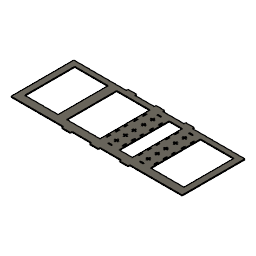
Plaat (Autodesk Fusion 360 design; units mm, degrees)
part number: 2026-03-19-08-41-09-141
Autodesk Fusion 360 part; units mm, degrees
sketch "Sketch1" plane through (0, 0, 0) normal (0, 0, 1) x (1, 0, 0)
  line L0 (-877.2181, -324.1666) -> (-877.2181, 35.8334)
  line L1 (-301.7378, 5.8334) -> (-226.7378, 5.8334)
  line L2 (-226.7378, 5.8334) -> (-226.7378, -279.1666)
  line L3 (-226.7378, -279.1666) -> (-301.7378, -279.1666)
  line L4 (-301.7378, -279.1666) -> (-301.7378, 5.8334)
  line L5 (-122.2181, 5.8334) -> (-122.2181, -279.1666)
  line L6 (67.7819, 5.8334) -> (-122.2181, 5.8334)
  line L7 (-652.2181, -279.1666) -> (-652.2181, 5.8334)
  line L8 (-842.2181, -279.1666) -> (-652.2181, -279.1666)
  line L9 (-652.2181, 5.8334) -> (-842.2181, 5.8334)
  line L10 (-842.2181, 5.8334) -> (-842.2181, -279.1666)
  line L11 (-412.2181, -279.1666) -> (-412.2181, 5.8334)
  line L12 (-602.2181, 5.8334) -> (-602.2181, -279.1666)
  line L13 (102.7819, 35.8334) -> (102.7819, -324.1666)
  line L14 (-358.9778, -149.6866) -> (-354.9778, -149.6866)
  line L15 (-354.9778, -129.6866) -> (-358.9778, -129.6866)
  line L16 (-366.9778, -137.6866) -> (-366.9778, -141.6866)
  line L17 (-358.9778, -137.6866) -> (-366.9778, -137.6866)
  line L18 (-346.9778, -137.6866) -> (-354.9778, -137.6866)
  line L19 (-358.9778, -141.6866) -> (-358.9778, -149.6866)
  line L20 (-354.9778, -149.6866) -> (-354.9778, -141.6866)
  line L21 (-366.9778, -141.6866) -> (-358.9778, -141.6866)
  line L22 (-346.9778, -141.6866) -> (-346.9778, -137.6866)
  line L23 (-358.9778, -129.6866) -> (-358.9778, -137.6866)
  line L24 (-354.9778, -137.6866) -> (-354.9778, -129.6866)
  line L25 (-354.9778, -141.6866) -> (-346.9778, -141.6866)
  line L26 (-354.9778, -31.3266) -> (-354.9778, -23.3266)
  line L27 (-346.9778, -35.3266) -> (-346.9778, -31.3266)
  line L28 (-354.9778, -43.3266) -> (-354.9778, -35.3266)
  line L29 (-358.9778, -31.3266) -> (-366.9778, -31.3266)
  line L30 (-358.9778, -23.3266) -> (-358.9778, -31.3266)
  line L31 (-358.9778, -35.3266) -> (-358.9778, -43.3266)
  line L32 (-358.9778, -43.3266) -> (-354.9778, -43.3266)
  line L33 (-346.9778, -31.3266) -> (-354.9778, -31.3266)
  line L34 (-354.9778, -23.3266) -> (-358.9778, -23.3266)
  line L35 (-366.9778, -35.3266) -> (-358.9778, -35.3266)
  line L36 (-354.9778, -35.3266) -> (-346.9778, -35.3266)
  line L37 (-366.9778, -31.3266) -> (-366.9778, -35.3266)
  line L38 (-358.9778, -94.4866) -> (-354.9778, -94.4866)
  line L39 (-354.9778, -82.4866) -> (-354.9778, -74.4866)
  line L40 (-354.9778, -74.4866) -> (-358.9778, -74.4866)
  line L41 (-354.9778, -86.4866) -> (-346.9778, -86.4866)
  line L42 (-346.9778, -86.4866) -> (-346.9778, -82.4866)
  line L43 (-358.9778, -86.4866) -> (-358.9778, -94.4866)
  line L44 (-366.9778, -86.4866) -> (-358.9778, -86.4866)
  line L45 (-366.9778, -82.4866) -> (-366.9778, -86.4866)
  line L46 (-354.9778, -94.4866) -> (-354.9778, -86.4866)
  line L47 (-346.9778, -82.4866) -> (-354.9778, -82.4866)
  line L48 (-358.9778, -82.4866) -> (-366.9778, -82.4866)
  line L49 (-358.9778, -74.4866) -> (-358.9778, -82.4866)
  line L50 (-358.9778, -238.0066) -> (-366.9778, -238.0066)
  line L51 (-354.9778, -238.0066) -> (-354.9778, -230.0066)
  line L52 (-366.9778, -238.0066) -> (-366.9778, -242.0066)
  line L53 (-354.9778, -242.0066) -> (-346.9778, -242.0066)
  line L54 (-358.9778, -230.0066) -> (-358.9778, -238.0066)
  line L55 (-358.9778, -242.0066) -> (-358.9778, -250.0066)
  line L56 (-358.9778, -250.0066) -> (-354.9778, -250.0066)
  line L57 (-346.9778, -242.0066) -> (-346.9778, -238.0066)
  line L58 (-346.9778, -238.0066) -> (-354.9778, -238.0066)
  line L59 (-366.9778, -242.0066) -> (-358.9778, -242.0066)
  line L60 (-354.9778, -250.0066) -> (-354.9778, -242.0066)
  line L61 (-354.9778, -230.0066) -> (-358.9778, -230.0066)
  line L62 (-354.9778, -190.8466) -> (-346.9778, -190.8466)
  line L63 (-366.9778, -186.8466) -> (-366.9778, -190.8466)
  line L64 (-358.9778, -190.8466) -> (-358.9778, -198.8466)
  line L65 (-358.9778, -198.8466) -> (-354.9778, -198.8466)
  line L66 (-354.9778, -186.8466) -> (-354.9778, -178.8466)
  line L67 (-346.9778, -186.8466) -> (-354.9778, -186.8466)
  line L68 (-358.9778, -186.8466) -> (-366.9778, -186.8466)
  line L69 (-366.9778, -190.8466) -> (-358.9778, -190.8466)
  line L70 (-354.9778, -178.8466) -> (-358.9778, -178.8466)
  line L71 (-346.9778, -190.8466) -> (-346.9778, -186.8466)
  line L72 (-354.9778, -198.8466) -> (-354.9778, -190.8466)
  line L73 (-358.9778, -178.8466) -> (-358.9778, -186.8466)
  line L74 (-356.9778, -139.6866) -> (-357.8185, -139.6866) construction
  line L75 (-357.8185, -139.6866) -> (-358.9778, -139.6866) construction
  line L76 (-602.2181, -279.1666) -> (-580.1685, -279.1666)
  line L77 (-580.1685, -279.1666) -> (-412.2181, -279.1666)
  line L78 (-602.2181, 5.8334) -> (-412.2181, 5.8334)
  line L79 (-122.2181, -279.1666) -> (67.7819, -279.1666)
  line L80 (67.7819, -279.1666) -> (67.7819, 5.8334)
  line L81 (-527.2181, 35.8334) -> (-527.2181, 45.8334)
  line L82 (-527.2181, 45.8334) -> (-577.2181, 45.8334)
  line L83 (-577.2181, 45.8334) -> (-577.2181, 35.8334)
  line L84 (-400.2181, -23.3266) -> (-404.2181, -23.3266)
  line L85 (-404.2181, -23.3266) -> (-404.2181, -43.3266)
  line L86 (-404.2181, -43.3266) -> (-400.2181, -43.3266)
  line L87 (-400.2181, -43.3266) -> (-400.2181, -23.3266)
  line L88 (-400.2181, -74.4866) -> (-404.2181, -74.4866)
  line L89 (-404.2181, -74.4866) -> (-404.2181, -94.4866)
  line L90 (-404.2181, -94.4866) -> (-400.2181, -94.4866)
  line L91 (-400.2181, -94.4866) -> (-400.2181, -74.4866)
  line L92 (-400.2181, -132.7485) -> (-404.2181, -132.7485)
  line L93 (-404.2181, -132.7485) -> (-404.2181, -149.6866)
  line L94 (-404.2181, -149.6866) -> (-400.2181, -149.6866)
  line L95 (-400.2181, -149.6866) -> (-400.2181, -132.7485)
  line L96 (-400.2181, -178.8466) -> (-404.2181, -178.8466)
  line L97 (-404.2181, -178.8466) -> (-404.2181, -198.8466)
  line L98 (-404.2181, -198.8466) -> (-400.2181, -198.8466)
  line L99 (-400.2181, -198.8466) -> (-400.2181, -178.8466)
  line L100 (-400.2181, -230.0066) -> (-404.2181, -230.0066)
  line L101 (-404.2181, -230.0066) -> (-404.2181, -250.0066)
  line L102 (-404.2181, -250.0066) -> (-400.2181, -250.0066)
  line L103 (-400.2181, -250.0066) -> (-400.2181, -230.0066)
  line L104 (-309.7378, -230.0066) -> (-313.7378, -230.0066)
  line L105 (-313.7378, -230.0066) -> (-313.7378, -250.0066)
  line L106 (-313.7378, -250.0066) -> (-309.7378, -250.0066)
  line L107 (-309.7378, -250.0066) -> (-309.7378, -230.0066)
  line L108 (-309.7378, -178.8466) -> (-313.7378, -178.8466)
  line L109 (-313.7378, -178.8466) -> (-313.7378, -198.8466)
  line L110 (-313.7378, -198.8466) -> (-309.7378, -198.8466)
  line L111 (-309.7378, -198.8466) -> (-309.7378, -178.8466)
  line L112 (-309.7378, -132.7485) -> (-313.7378, -132.7485)
  line L113 (-313.7378, -132.7485) -> (-313.7378, -149.6866)
  line L114 (-313.7378, -149.6866) -> (-309.7378, -149.6866)
  line L115 (-309.7378, -149.6866) -> (-309.7378, -132.7485)
  line L116 (-309.7378, -74.4866) -> (-313.7378, -74.4866)
  line L117 (-313.7378, -74.4866) -> (-313.7378, -94.4866)
  line L118 (-313.7378, -94.4866) -> (-309.7378, -94.4866)
  line L119 (-309.7378, -94.4866) -> (-309.7378, -74.4866)
  line L120 (-309.7378, -23.3266) -> (-313.7378, -23.3266)
  line L121 (-313.7378, -23.3266) -> (-313.7378, -43.3266)
  line L122 (-313.7378, -43.3266) -> (-309.7378, -43.3266)
  line L123 (-309.7378, -43.3266) -> (-309.7378, -23.3266)
  line L124 (-197.2181, 35.8334) -> (-197.2181, 45.8334)
  line L125 (-197.2181, 45.8334) -> (-247.2181, 45.8334)
  line L126 (-247.2181, 45.8334) -> (-247.2181, 35.8334)
  line L127 (-367.2181, 35.8334) -> (-367.2181, 45.8334)
  line L128 (-367.2181, 45.8334) -> (-417.2181, 45.8334)
  line L129 (-417.2181, 45.8334) -> (-417.2181, 35.8334)
  line L130 (-877.2181, 35.8334) -> (-577.2181, 35.8334)
  line L131 (-527.2181, 35.8334) -> (-417.2181, 35.8334)
  line L132 (-367.2181, 35.8334) -> (-247.2181, 35.8334)
  line L133 (-197.2181, 35.8334) -> (102.7819, 35.8334)
  line L134 (-366.9778, -279.1666) -> (-346.9778, -279.1666)
  line L135 (-346.9778, -279.1666) -> (-346.9778, -275.1666)
  line L136 (-346.9778, -275.1666) -> (-366.9778, -275.1666)
  line L137 (-366.9778, -275.1666) -> (-366.9778, -279.1666)
  line L138 (-366.9778, 5.8334) -> (-346.9778, 5.8334)
  line L139 (-346.9778, 5.8334) -> (-346.9778, 1.8334)
  line L140 (-346.9778, 1.8334) -> (-366.9778, 1.8334)
  line L141 (-366.9778, 1.8334) -> (-366.9778, 5.8334)
  line L142 (-527.2181, -324.1666) -> (-527.2181, -334.1666)
  line L143 (-527.2181, -334.1666) -> (-577.2181, -334.1666)
  line L144 (-577.2181, -334.1666) -> (-577.2181, -324.1666)
  line L145 (-367.2181, -324.1666) -> (-367.2181, -334.1666)
  line L146 (-367.2181, -334.1666) -> (-417.2181, -334.1666)
  line L147 (-417.2181, -334.1666) -> (-417.2181, -324.1666)
  line L148 (-197.2181, -324.1666) -> (-197.2181, -334.1666)
  line L149 (-197.2181, -334.1666) -> (-247.2181, -334.1666)
  line L150 (-247.2181, -334.1666) -> (-247.2181, -324.1666)
  line L151 (-877.2181, -324.1666) -> (-577.2181, -324.1666)
  line L152 (-527.2181, -324.1666) -> (-417.2181, -324.1666)
  line L153 (-367.2181, -324.1666) -> (-247.2181, -324.1666)
  line L154 (-197.2181, -324.1666) -> (102.7819, -324.1666)
  line L155 (-127.7378, -178.8466) -> (-131.7378, -178.8466)
  line L156 (-127.7378, -250.0066) -> (-127.7378, -230.0066)
  line L157 (-127.7378, -198.8466) -> (-127.7378, -178.8466)
  line L158 (-131.7378, -198.8466) -> (-127.7378, -198.8466)
  line L159 (-131.7378, -230.0066) -> (-131.7378, -250.0066)
  line L160 (-131.7378, -178.8466) -> (-131.7378, -198.8466)
  line L161 (-127.7378, -230.0066) -> (-131.7378, -230.0066)
  line L162 (-131.7378, -250.0066) -> (-127.7378, -250.0066)
  line L163 (-127.7378, -149.6866) -> (-127.7378, -132.7485)
  line L164 (-127.7378, -94.4866) -> (-127.7378, -74.4866)
  line L165 (-131.7378, -132.7485) -> (-131.7378, -149.6866)
  line L166 (-131.7378, -74.4866) -> (-131.7378, -94.4866)
  line L167 (-127.7378, -74.4866) -> (-131.7378, -74.4866)
  line L168 (-127.7378, -132.7485) -> (-131.7378, -132.7485)
  line L169 (-131.7378, -149.6866) -> (-127.7378, -149.6866)
  line L170 (-131.7378, -94.4866) -> (-127.7378, -94.4866)
  line L171 (-127.7378, -43.3266) -> (-127.7378, -23.3266)
  line L172 (-131.7378, -23.3266) -> (-131.7378, -43.3266)
  line L173 (-131.7378, -43.3266) -> (-127.7378, -43.3266)
  line L174 (-127.7378, -23.3266) -> (-131.7378, -23.3266)
  line L175 (-184.9778, -279.1666) -> (-164.9778, -279.1666)
  line L176 (-172.9778, -198.8466) -> (-172.9778, -190.8466)
  line L177 (-218.2181, -132.7485) -> (-222.2181, -132.7485)
  line L178 (-184.9778, -190.8466) -> (-176.9778, -190.8466)
  line L179 (-184.9778, -186.8466) -> (-184.9778, -190.8466)
  line L180 (-175.8185, -139.6866) -> (-176.9778, -139.6866) construction
  line L181 (-164.9778, -279.1666) -> (-164.9778, -275.1666)
  line L182 (-172.9778, -149.6866) -> (-172.9778, -141.6866)
  line L183 (-176.9778, -242.0066) -> (-176.9778, -250.0066)
  line L184 (-172.9778, -230.0066) -> (-176.9778, -230.0066)
  line L185 (-218.2181, -178.8466) -> (-222.2181, -178.8466)
  line L186 (-184.9778, -275.1666) -> (-184.9778, -279.1666)
  line L187 (-176.9778, -82.4866) -> (-184.9778, -82.4866)
  line L188 (-176.9778, -137.6866) -> (-184.9778, -137.6866)
  line L189 (-172.9778, -250.0066) -> (-172.9778, -242.0066)
  line L190 (-172.9778, -190.8466) -> (-164.9778, -190.8466)
  line L191 (-218.2181, -230.0066) -> (-222.2181, -230.0066)
  line L192 (-164.9778, -141.6866) -> (-164.9778, -137.6866)
  line L193 (-172.9778, -178.8466) -> (-176.9778, -178.8466)
  line L194 (-164.9778, -86.4866) -> (-164.9778, -82.4866)
  line L195 (-222.2181, -178.8466) -> (-222.2181, -198.8466)
  line L196 (-164.9778, -275.1666) -> (-184.9778, -275.1666)
  line L197 (-164.9778, -242.0066) -> (-164.9778, -238.0066)
  line L198 (-218.2181, -149.6866) -> (-218.2181, -132.7485)
  line L199 (-164.9778, 1.8334) -> (-184.9778, 1.8334)
  line L200 (-164.9778, -31.3266) -> (-172.9778, -31.3266)
  line L201 (-184.9778, -35.3266) -> (-176.9778, -35.3266)
  line L202 (-172.9778, -137.6866) -> (-172.9778, -129.6866)
  line L203 (-184.9778, -82.4866) -> (-184.9778, -86.4866)
  line L204 (-164.9778, -82.4866) -> (-172.9778, -82.4866)
  line L205 (-222.2181, -94.4866) -> (-218.2181, -94.4866)
  line L206 (-172.9778, -74.4866) -> (-176.9778, -74.4866)
  line L207 (-222.2181, -74.4866) -> (-222.2181, -94.4866)
  line L208 (-172.9778, -94.4866) -> (-172.9778, -86.4866)
  line L209 (-164.9778, -137.6866) -> (-172.9778, -137.6866)
  line L210 (-164.9778, -35.3266) -> (-164.9778, -31.3266)
  line L211 (-176.9778, -35.3266) -> (-176.9778, -43.3266)
  line L212 (-172.9778, -82.4866) -> (-172.9778, -74.4866)
  line L213 (-172.9778, -86.4866) -> (-164.9778, -86.4866)
  line L214 (-184.9778, 5.8334) -> (-164.9778, 5.8334)
  line L215 (-218.2181, -43.3266) -> (-218.2181, -23.3266)
  line L216 (-164.9778, 5.8334) -> (-164.9778, 1.8334)
  line L217 (-176.9778, -129.6866) -> (-176.9778, -137.6866)
  line L218 (-176.9778, -31.3266) -> (-184.9778, -31.3266)
  line L219 (-184.9778, -141.6866) -> (-176.9778, -141.6866)
  line L220 (-184.9778, -31.3266) -> (-184.9778, -35.3266)
  line L221 (-176.9778, -23.3266) -> (-176.9778, -31.3266)
  line L222 (-172.9778, -129.6866) -> (-176.9778, -129.6866)
  line L223 (-176.9778, -94.4866) -> (-172.9778, -94.4866)
  line L224 (-164.9778, -190.8466) -> (-164.9778, -186.8466)
  line L225 (-164.9778, -238.0066) -> (-172.9778, -238.0066)
  line L226 (-172.9778, -35.3266) -> (-164.9778, -35.3266)
  line L227 (-222.2181, -132.7485) -> (-222.2181, -149.6866)
  line L228 (-172.9778, -186.8466) -> (-172.9778, -178.8466)
  line L229 (-222.2181, -198.8466) -> (-218.2181, -198.8466)
  line L230 (-184.9778, -86.4866) -> (-176.9778, -86.4866)
  line L231 (-184.9778, -137.6866) -> (-184.9778, -141.6866)
  line L232 (-172.9778, -141.6866) -> (-164.9778, -141.6866)
  line L233 (-218.2181, -23.3266) -> (-222.2181, -23.3266)
  line L234 (-184.9778, 1.8334) -> (-184.9778, 5.8334)
  line L235 (-172.9778, -242.0066) -> (-164.9778, -242.0066)
  line L236 (-176.9778, -149.6866) -> (-172.9778, -149.6866)
  line L237 (-184.9778, -238.0066) -> (-184.9778, -242.0066)
  line L238 (-222.2181, -250.0066) -> (-218.2181, -250.0066)
  line L239 (-176.9778, -178.8466) -> (-176.9778, -186.8466)
  line L240 (-222.2181, -230.0066) -> (-222.2181, -250.0066)
  line L241 (-172.9778, -31.3266) -> (-172.9778, -23.3266)
  line L242 (-176.9778, -190.8466) -> (-176.9778, -198.8466)
  line L243 (-176.9778, -141.6866) -> (-176.9778, -149.6866)
  line L244 (-172.9778, -238.0066) -> (-172.9778, -230.0066)
  line L245 (-176.9778, -250.0066) -> (-172.9778, -250.0066)
  line L246 (-176.9778, -186.8466) -> (-184.9778, -186.8466)
  line L247 (-174.9778, -139.6866) -> (-175.8185, -139.6866) construction
  line L248 (-164.9778, -186.8466) -> (-172.9778, -186.8466)
  line L249 (-172.9778, -43.3266) -> (-172.9778, -35.3266)
  line L250 (-172.9778, -23.3266) -> (-176.9778, -23.3266)
  line L251 (-176.9778, -86.4866) -> (-176.9778, -94.4866)
  line L252 (-184.9778, -242.0066) -> (-176.9778, -242.0066)
  line L253 (-218.2181, -198.8466) -> (-218.2181, -178.8466)
  line L254 (-176.9778, -238.0066) -> (-184.9778, -238.0066)
  line L255 (-218.2181, -250.0066) -> (-218.2181, -230.0066)
  line L256 (-176.9778, -43.3266) -> (-172.9778, -43.3266)
  line L257 (-176.9778, -198.8466) -> (-172.9778, -198.8466)
  line L258 (-218.2181, -94.4866) -> (-218.2181, -74.4866)
  line L259 (-222.2181, -149.6866) -> (-218.2181, -149.6866)
  line L260 (-176.9778, -230.0066) -> (-176.9778, -238.0066)
  line L261 (-176.9778, -74.4866) -> (-176.9778, -82.4866)
  line L262 (-218.2181, -74.4866) -> (-222.2181, -74.4866)
  line L263 (-222.2181, -43.3266) -> (-218.2181, -43.3266)
  line L264 (-222.2181, -23.3266) -> (-222.2181, -43.3266)
  point P0 (-356.9778, -139.6866)
  point P1 (-358.9778, -139.6866)
  point P2 (-174.9778, -139.6866)
  point P3 (-176.9778, -139.6866)
  constraint vertical L11
  constraint horizontal L14
  constraint perpendicular L14 L20
  constraint perpendicular L20 L25
  constraint perpendicular L22 L25
  constraint perpendicular L18 L22
  constraint perpendicular L18 L24
  constraint perpendicular L15 L24
  constraint perpendicular L18 L23
  constraint perpendicular L17 L23
  constraint perpendicular L16 L17
  constraint perpendicular L16 L21
  constraint perpendicular L19 L21
  constraint horizontal L32
  constraint perpendicular L28 L32
  constraint perpendicular L28 L36
  constraint perpendicular L27 L36
  constraint perpendicular L27 L33
  constraint perpendicular L26 L33
  constraint perpendicular L26 L34
  constraint perpendicular L30 L33
  constraint perpendicular L29 L30
  constraint perpendicular L29 L37
  constraint perpendicular L35 L37
  constraint perpendicular L31 L35
  constraint horizontal L38
  constraint perpendicular L38 L46
  constraint perpendicular L41 L46
  constraint perpendicular L41 L42
  constraint perpendicular L42 L47
  constraint perpendicular L39 L47
  constraint perpendicular L39 L40
  constraint perpendicular L47 L49
  constraint perpendicular L48 L49
  constraint perpendicular L45 L48
  constraint perpendicular L44 L45
  constraint perpendicular L43 L44
  constraint horizontal L56
  constraint perpendicular L56 L60
  constraint perpendicular L53 L60
  constraint perpendicular L53 L57
  constraint perpendicular L57 L58
  constraint perpendicular L51 L58
  constraint perpendicular L51 L61
  constraint perpendicular L54 L58
  constraint perpendicular L50 L54
  constraint perpendicular L50 L52
  constraint perpendicular L52 L59
  constraint perpendicular L55 L59
  constraint horizontal L65
  constraint perpendicular L65 L72
  constraint perpendicular L62 L72
  constraint perpendicular L62 L71
  constraint perpendicular L67 L71
  constraint perpendicular L66 L67
  constraint perpendicular L66 L70
  constraint perpendicular L67 L73
  constraint perpendicular L68 L73
  constraint perpendicular L63 L68
  constraint perpendicular L63 L69
  constraint perpendicular L64 L69
  constraint coincident P0 L74.start
  constraint coincident P1 L75.end
  constraint perpendicular L12 L76
  constraint perpendicular L11 L77
  constraint perpendicular L11 L78
  constraint perpendicular L5 L79
  constraint perpendicular L6 L80
  constraint vertical L81
  constraint horizontal L82
  constraint vertical L83
  constraint horizontal L84
  constraint vertical L85
  constraint horizontal L86
  constraint vertical L87
  constraint horizontal L88
  constraint vertical L89
  constraint horizontal L90
  constraint vertical L91
  constraint horizontal L92
  constraint vertical L93
  constraint horizontal L94
  constraint vertical L95
  constraint horizontal L96
  constraint vertical L97
  constraint horizontal L98
  constraint vertical L99
  constraint horizontal L100
  constraint vertical L101
  constraint horizontal L102
  constraint vertical L103
  constraint horizontal L104
  constraint vertical L105
  constraint horizontal L106
  constraint vertical L107
  constraint horizontal L108
  constraint vertical L109
  constraint horizontal L110
  constraint vertical L111
  constraint horizontal L112
  constraint vertical L113
  constraint horizontal L114
  constraint vertical L115
  constraint horizontal L116
  constraint vertical L117
  constraint horizontal L118
  constraint vertical L119
  constraint horizontal L120
  constraint vertical L121
  constraint horizontal L122
  constraint vertical L123
  constraint vertical L124
  constraint horizontal L125
  constraint vertical L126
  constraint vertical L127
  constraint horizontal L128
  constraint vertical L129
  constraint perpendicular L83 L130
  constraint perpendicular L129 L131
  constraint perpendicular L126 L132
  constraint perpendicular L13 L133
  constraint horizontal L134
  constraint vertical L135
  constraint horizontal L136
  constraint vertical L137
  constraint horizontal L138
  constraint vertical L139
  constraint horizontal L140
  constraint vertical L141
  constraint vertical L142
  constraint horizontal L143
  constraint vertical L144
  constraint vertical L145
  constraint horizontal L146
  constraint vertical L147
  constraint vertical L148
  constraint horizontal L149
  constraint vertical L150
  constraint perpendicular L150 L153
  constraint perpendicular L13 L154
  constraint horizontal L236
  constraint perpendicular L182 L236
  constraint perpendicular L182 L232
  constraint perpendicular L192 L232
  constraint perpendicular L192 L209
  constraint perpendicular L202 L209
  constraint perpendicular L202 L222
  constraint perpendicular L209 L217
  constraint perpendicular L188 L217
  constraint perpendicular L188 L231
  constraint perpendicular L219 L231
  constraint perpendicular L219 L243
  constraint horizontal L256
  constraint perpendicular L249 L256
  constraint perpendicular L226 L249
  constraint perpendicular L210 L226
  constraint perpendicular L200 L210
  constraint perpendicular L200 L241
  constraint perpendicular L241 L250
  constraint perpendicular L200 L221
  constraint perpendicular L218 L221
  constraint perpendicular L218 L220
  constraint perpendicular L201 L220
  constraint perpendicular L201 L211
  constraint horizontal L223
  constraint perpendicular L208 L223
  constraint perpendicular L208 L213
  constraint perpendicular L194 L213
  constraint perpendicular L194 L204
  constraint perpendicular L204 L212
  constraint perpendicular L206 L212
  constraint perpendicular L204 L261
  constraint perpendicular L187 L261
  constraint perpendicular L187 L203
  constraint perpendicular L203 L230
  constraint perpendicular L230 L251
  constraint horizontal L245
  constraint perpendicular L189 L245
  constraint perpendicular L189 L235
  constraint perpendicular L197 L235
  constraint perpendicular L197 L225
  constraint perpendicular L225 L244
  constraint perpendicular L184 L244
  constraint perpendicular L225 L260
  constraint perpendicular L254 L260
  constraint perpendicular L237 L254
  constraint perpendicular L237 L252
  constraint perpendicular L183 L252
  constraint horizontal L257
  constraint perpendicular L176 L257
  constraint perpendicular L176 L190
  constraint perpendicular L190 L224
  constraint perpendicular L224 L248
  constraint perpendicular L228 L248
  constraint perpendicular L193 L228
  constraint perpendicular L239 L248
  constraint perpendicular L239 L246
  constraint perpendicular L179 L246
  constraint perpendicular L178 L179
  constraint perpendicular L178 L242
  constraint coincident P2 L247.start
  constraint coincident P3 L180.end
  constraint horizontal L233
  constraint vertical L264
  constraint horizontal L263
  constraint vertical L215
  constraint horizontal L262
  constraint vertical L207
  constraint horizontal L205
  constraint vertical L258
  constraint horizontal L177
  constraint vertical L227
  constraint horizontal L259
  constraint vertical L198
  constraint horizontal L185
  constraint vertical L195
  constraint horizontal L229
  constraint vertical L253
  constraint horizontal L191
  constraint vertical L240
  constraint horizontal L238
  constraint vertical L255
  constraint horizontal L161
  constraint vertical L159
  constraint horizontal L162
  constraint vertical L156
  constraint horizontal L155
  constraint vertical L160
  constraint horizontal L158
  constraint vertical L157
  constraint horizontal L168
  constraint vertical L165
  constraint horizontal L169
  constraint vertical L163
  constraint horizontal L167
  constraint vertical L166
  constraint horizontal L170
  constraint vertical L164
  constraint horizontal L174
  constraint vertical L172
  constraint horizontal L173
  constraint vertical L171
  constraint horizontal L175
  constraint vertical L181
  constraint horizontal L196
  constraint vertical L186
  constraint horizontal L214
  constraint vertical L216
  constraint horizontal L199
  constraint vertical L234
extrude "Extrude4" add sketch "Sketch1" along normal blind 4
equation "d9 = 40 mm"
equation "d11 = d9"
equation "d13 = d79"
equation "d79 = 45 mm"
equation "d113 = 8 mm"
equation "d116 = d113"
